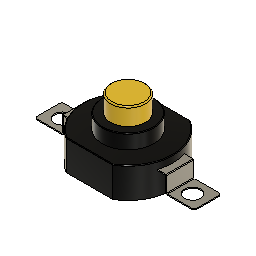
2Pin Horizontal Flashlight Button Switch 1412-KD Self Lock ON-OFF SPST Yellow v8 (Autodesk Fusion 360 design; units mm, degrees)
Autodesk Fusion 360 part; units mm, degrees
sketch "Sketch1" plane through (0, 0, 0) normal (0, 0, 1) x (1, 0, 0) in component "BodySw"
  circle A0 centre (0, 0) radius 4
  circle A1 centre (0, 0) radius 7
  line L0 (-6, 6) -> (6, 6)
  line L1 (6, 6) -> (6, -6) construction
  line L2 (6, -6) -> (-6, -6)
  line L3 (-6, -6) -> (-6, 6) construction
  line L4 (-6, 6) -> (6, -6) construction
  line L5 (6, 6) -> (-6, -6) construction
  dimension "d1" = 8
  dimension "d2" = 14
  dimension "d3" = 12
  dimension "d4" = 12
  constraint coincident A0.centre A1.centre
  constraint horizontal L0
  constraint vertical L1
  constraint horizontal L2
  constraint vertical L3
  constraint coincident A0.centre L5
  constraint coincident A0.centre L4
  measures "d1" diameter of A0
  measures "d2" diameter of A1
  measures "d3" distance of L0.start L0.end
  measures "d4" distance of L0.start L2.end
extrude "Extrude2" add sketch "Sketch1" along normal blind 4.7 contours A0 | A1 L0 L2 makes body 1 in component "BodySw"
extrude "Extrude3" add sketch "Sketch1" along normal blind 6.9 contours A0 bodies 1 in component "BodySw"
fillet "Fillet1" radius 0.1 5 edges at (0, -6, 4.7) (7, 0, 4.7) (0, 6, 4.7) (-7, 0, 4.7) (-3.7293, -1.4465, 6.9) on bodies 1 in component "BodySw"
sketch "Sketch1 (2)" plane through (0, 0, 6.9) normal (0, 0, 1) x (1, 0, 0) in component "SwBotton"
  circle A0 centre (0, 0) radius 2.7
  circle A1 centre (0, 0) radius 3.9
  dimension "d12" = 5.4
  constraint coincident A0.centre A1.centre
  measures "d12" diameter of A0
extrude "Extrude1" add sketch "Sketch1 (2)" along normal blind 2.7 separate body contours A0 makes body 2 in component "SwBotton"
fillet "Fillet1'" radius 0.2 1 edges at (-2.5173, -0.9764, 9.6) on bodies 2 in component "SwBotton"
ref_plane "WorkPlane1" through (0, 0, 0.9) normal (0, 0, 1) x (1, 0, 0) in component "ContactPins"
sketch "Sketch1 (3)" plane through (0, 0, 0.9) normal (0, 0, 1) x (1, 0, 0) in component "ContactPins"
  line L0 (7.96, -2.1) -> (-7.96, -2.1)
  line L1 (-7.96, -2.1) -> (-7.96, 2.1)
  line L2 (-7.96, 2.1) -> (7.96, 2.1)
  line L3 (7.96, 2.1) -> (7.96, -2.1)
  line L4 (7.96, -2.1) -> (-7.96, 2.1) construction
  line L5 (-7.96, -2.1) -> (7.96, 2.1) construction
  line L6 (12.4, -2.1) -> (-12.4, -2.1)
  line L7 (-12.4, -2.1) -> (-12.4, 2.1)
  line L8 (-12.4, 2.1) -> (12.4, 2.1)
  line L9 (12.4, 2.1) -> (12.4, -2.1)
  line L10 (12.4, -2.1) -> (-12.4, 2.1) construction
  line L11 (-12.4, -2.1) -> (12.4, 2.1) construction
  dimension "d21" = 15.92
  dimension "d22" = 4.2
  dimension "d23" = 24.8
  dimension "d24" = 4.2
  constraint perpendicular L0 L1
  constraint parallel L0 L2
  constraint parallel L1 L3
  constraint horizontal L0
  constraint coincident L4 origin
  constraint coincident L5 origin
  constraint perpendicular L6 L7
  constraint parallel L6 L8
  constraint parallel L7 L9
  constraint horizontal L6
  constraint coincident L10 origin
  constraint coincident L11 origin
  measures "d21" distance of L1.end L2.end
  measures "d22" distance of L0.end L1.end
  measures "d23" distance of L7.end L8.end
  measures "d24" distance of L6.end L7.end
extrude "Extrude1'" add sketch "Sketch1 (3)" along normal blind 0.16 separate body contours L3 L6 L8 L9 makes body 3 in component "ContactPins"
hole "Hole1" at (10.1204, -0.0779, 1.06) direction (0, 0, -1) diameter 2.5 depth 2 tip angle 118 bodies 3 in component "ContactPins"
sketch "Sketch2" plane through (0, 0, 1.06) normal (0, 0, 1) x (-1, 0, 0) in component "ContactPins"
  circle A0 centre (-10.1204, 0.0779) radius 1.25
  line L0 (-7.96, -2.1) -> (-7.96, 2.1)
  line L1 (-7.96, 2.1) -> (-12.4, 2.1)
  line L2 (-12.4, 2.1) -> (-12.4, -2.1)
  line L3 (-12.4, -2.1) -> (-7.96, -2.1)
  line L4 (-7.96, -2.1) -> (-8.12, -2.1)
  line L5 (-8.12, -2.1) -> (-8.12, 2.1)
  line L6 (-8.12, 2.1) -> (-7.96, 2.1)
  line L7 (-7.96, 2.1) -> (-7.96, -2.1)
  dimension "d30" = 0.16
  constraint horizontal L4
  constraint vertical L5
  constraint horizontal L6
  constraint vertical L7
  constraint coincident L0.start L3.end
  measures "d30" distance of L0.start L4.end
extrude "Extrude2'" add sketch "Sketch2" along normal blind 2.56 contours L0 L1 L3 L4 L5 L6 L7 bodies 3 in component "ContactPins"
sketch "Sketch3" plane through (7.96, 0, 0) normal (-1, 0, 0) x (0, -1, 0) in component "ContactPins"
  line L0 (-2.1, 0.9) -> (2.1, 0.9)
  line L1 (2.1, 0.9) -> (2.1, 3.62)
  line L2 (2.1, 3.62) -> (-2.1, 3.62)
  line L3 (-2.1, 3.62) -> (-2.1, 0.9)
  line L4 (-2.1, 3.62) -> (2.1, 3.62)
  line L5 (2.1, 3.62) -> (2.1, 3.46)
  line L6 (2.1, 3.46) -> (-2.1, 3.46)
  line L7 (-2.1, 3.46) -> (-2.1, 3.62)
  dimension "d33" = 0.16
  constraint horizontal L4
  constraint vertical L5
  constraint horizontal L6
  constraint vertical L7
  constraint coincident L2.end L3.start
  measures "d33" distance of L2.end L6.end
extrude "Extrude3'" add sketch "Sketch3" along normal up to surface contours L1 L2 L3 L4 L5 L6 L7 end surface at (4.1757, 5.6182, 1.5333) on bodies 1 bodies 3 in component "ContactPins"
fillet "Fillet1''" radius 0.1 4 edges at (8.12, 0, 3.62) (7.96, 0, 0.9) (7.96, 0, 3.46) (8.12, 0, 1.06) on bodies 3 in component "ContactPins"
fillet "Fillet2" radius 0.4 2 edges at (12.4, -2.1, 0.98) (12.4, 2.1, 0.98) on bodies 3 in component "ContactPins"
mirror "Mirror1" about plane through (0, 0, 0) normal (1, 0, 0) of bodies 3 makes body 4 in component "ContactPins"
sketch "Sketch2 (2)" plane through (0, 0, 0) normal (0, 0, -1) x (1, 0, 0) in component "BodySw"
  arc A0 (-3.6056, 6) -> (-3.6056, -6) centre (0, 0) ccw
  line L0 (-3.6056, -6) -> (3.6056, -6)
  arc A1 (3.6056, -6) -> (3.6056, 6) centre (0, 0) ccw
  line L1 (3.6056, 6) -> (-3.6056, 6)
  line L2 (-3.3654, 5.0757) -> (-3.3654, -5.258) construction
  line L3 (-3.3654, -5.258) -> (-1.6654, -5.258) construction
  line L4 (-1.6654, -5.258) -> (-1.6654, 5.0757) construction
  line L5 (-1.6654, 5.0757) -> (-3.3654, 5.0757) construction
  line L6 (-1.135, 3.3706) -> (-1.135, -3.3945) construction
  line L7 (-1.135, -3.3945) -> (0.565, -3.3945) construction
  line L8 (0.565, -3.3945) -> (0.565, 3.3706) construction
  line L9 (0.565, 3.3706) -> (-1.135, 3.3706) construction
  text T0 "1.5A 250V AC" font "Arial" height 1.7 align ink ink in box 0 x 0 at (-3.3654, 5.0757) x (0, -1) y (1, 0) spacing 1 kerned height is em
  text T1 "CNYTEN" font "Arial" height 1.7 align ink ink in box 0 x 0 at (-1.135, 3.3706) x (0, -1) y (1, 0) spacing 1 kerned height is em
  constraint perpendicular L2 L3
  constraint parallel L2 L4
  constraint parallel L3 L5
  constraint perpendicular L6 L7
  constraint parallel L6 L8
  constraint parallel L7 L9
extrude "Extrude4" cut sketch "Sketch2 (2)" against normal blind 0.1 text T1 T0 bodies 1 in component "BodySw"
component "BodySw" placed x (1, 0, 0) y (0, 1, 0) z (0, 0, 1) at (0, 0, 0)
component "SwBotton" placed x (1, 0, 0) y (0, 1, 0) z (0, 0, 1) at (0, 0, 0) in component "BodySw"
component "ContactPins" placed x (1, 0, 0) y (0, 1, 0) z (0, 0, 1) at (0, 0, 0) in component "SwBotton"
equation "d14 = 9.6 mm - 6.9 mm"
equation "d31 = 2.4 mm + 0.16 mm"
named bodies: "BodySw", "SwBotton", "ContactPins Right", "ContactPins Left"
